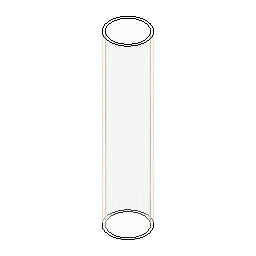
Clear Acrylic Tube v1 (Autodesk Fusion 360 design; units mm, degrees)
Autodesk Fusion 360 part; units mm, degrees
cylinder "CylinderPrimitive1" add diameter 177.8 height 814.3875 placed x (1, 0, 0) y (0, 1, 0) z (0, 0, 1) at (0, 0, 0)
sketch "Sketch2" plane through (0, 0, 0) normal (0, 0, 1) x (1, 0, 0)
  circle A0 centre (0, 0) radius 77.7875
  dimension "d3" = 155.575
  constraint coincident A0.centre origin
  measures "d3" diameter of A0
extrude "Extrude1" cut sketch "Sketch2" along normal blind 1016
equation "d1 = 32 1/16\""
